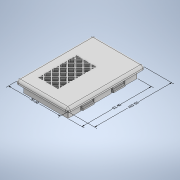
# Autodesk Inventor part: Part_A2
Saved by Autodesk Inventor 2022.6 (Build 266554010, 554A)
## iProperties
Created: 2025-05-14
Part Number: Part_A2
Material: Generic
Document SubType Name: Modeling
Designer: khinm
Density: 1 g/cm^3
Appearance: Default
Author: khinm
Autodesk Inventor part; units mm, degrees
ref_plane "YZ Plane" through (0, 0, 0) normal (1, 0, 0) x (0, 1, 0)
ref_plane "XZ Plane" through (0, 0, 0) normal (0, 1, 0) x (-1, 0, 0)
sketch "Sketch1" plane through (0, 0, 0) normal (0, 1, 0) x (-1, 0, 0)
  line L0 (35, -51.75) -> (-35, -51.75)
  line L1 (-35, -51.75) -> (-35, 51.75)
  line L2 (-35, 51.75) -> (35, 51.75)
  line L3 (35, 51.75) -> (35, -51.75)
  point P0 (0, 0)
  point P1 (35, 0)
  point P2 (0, -51.75)
  dimension "d0" = 70
  dimension "d1" = 103.5
  constraints: 8 end point, 2 midpoint, 2 parallel, 1 horizontal, 1 horizontal alignment, 1 perpendicular, 1 vertical alignment
  measures "d0" distance of L0.start L0.end
  measures "d1" distance of L0.end L1.end
extrude "Extrusion1" add sketch "Sketch1" along normal blind 5
sketch "Sketch2" plane through (0, 0, 0) normal (0, -1, 0) x (1, 0, 0)
  line L0 (-29.95, 46.7) -> (29.95, 46.7)
  line L1 (29.95, 46.7) -> (29.95, -46.7)
  line L2 (29.95, -46.7) -> (-29.95, -46.7)
  line L3 (-29.95, -46.7) -> (-29.95, 46.7)
  line L4 (-35, -51.75) -> (-35, 51.75) projected
  line L5 (-35, 51.75) -> (35, 51.75) projected
  point P0 (0, 0)
  point P1 (-29.95, 0)
  point P2 (-35, 0)
  point P3 (0, 46.7)
  point P4 (0, 51.75)
  dimension "d4" = 59.9
  dimension "d5" = 93.4
  constraints: 8 end point, 4 midpoint, 2 parallel, 1 horizontal, 1 horizontal alignment, 1 perpendicular, 1 vertical alignment
  measures "d4" distance of L0.start L0.end
  measures "d5" distance of L0.end L1.end
extrude "Extrusion2" add sketch "Sketch2" along normal blind 11
sketch "Sketch3" plane through (0, -11, 0) normal (0, -1, 0) x (1, 0, 0)
  line L0 (-28.45, 45.2) -> (28.45, 45.2)
  line L1 (28.45, 45.2) -> (28.45, -45.2)
  line L2 (28.45, -45.2) -> (-28.45, -45.2)
  line L3 (-28.45, -45.2) -> (-28.45, 45.2)
  line L4 (29.95, 46.7) -> (-29.95, 46.7) projected
  line L5 (-29.95, 46.7) -> (-29.95, -46.7) projected
  point P0 (0, 0)
  point P1 (0, 45.2)
  point P2 (0, 46.7)
  point P3 (-28.45, 0)
  dimension "d8" = 1.5
  dimension "d9" = 1.5
  constraints: 8 end point, 3 midpoint, 2 parallel, 2 vertical alignment, 1 horizontal, 1 horizontal alignment, 1 perpendicular
  measures "d8" distance between parallel lines of L4 L0
  measures "d9" distance between parallel lines of L5 L3
extrude "Extrusion3" cut sketch "Sketch3" against normal up to surface (11 mm away)
sketch "Sketch4" plane through (29.95, 0, 46.7) normal (1, 0, 0) x (0, 0, -1)
  line L0 (93.4, -11) -> (0, -11) projected
  line L1 (17.025, -2) -> (18.525, -2)
  line L2 (18.525, -2) -> (18.525, -11)
  line L3 (18.525, -11) -> (17.025, -11)
  line L4 (17.025, -11) -> (17.025, -2)
  line L5 (58.375, -2) -> (59.875, -2)
  line L6 (59.875, -2) -> (59.875, -11)
  line L7 (59.875, -11) -> (58.375, -11)
  line L8 (58.375, -11) -> (58.375, -2)
  line L9 (33.525, -2) -> (35.025, -2)
  line L10 (35.025, -2) -> (35.025, -11)
  line L11 (35.025, -11) -> (33.525, -11)
  line L12 (33.525, -11) -> (33.525, -2)
  line L13 (74.875, -2) -> (76.375, -2)
  line L14 (76.375, -2) -> (76.375, -11)
  line L15 (76.375, -11) -> (74.875, -11)
  line L16 (74.875, -11) -> (74.875, -2)
  line L17 (35.025, -11) -> (58.375, -11)
  line L18 (-5.05, 0) -> (98.45, 0) projected
  point P0 (46.7, 0)
  point P1 (46.7, 0)
  point P2 (46.7, -11)
  point P3 (17.025, -11)
  dimension "d12" = 1.5
  dimension "d13" = 9
  dimension "d14" = 1.5
  dimension "d15" = 9
  dimension "d16" = 9
  dimension "d17" = 1.5
  dimension "d18" = 1.5
  dimension "d19" = 23.35
  dimension "d20" = 15
  dimension "d21" = 15
  constraints: 34 end point, 8 parallel, 5 point on line, 4 horizontal, 4 perpendicular, 2 midpoint, 1 collinear, 1 vertical alignment
  measures "d12" distance of L1.start L1.end
  measures "d13" distance of L1.end L2.end
  measures "d14" distance between parallel lines of L6 L8
  measures "d15" distance of L9.end L10.end
  measures "d16" distance of L13.end L14.end
  measures "d17" distance between parallel lines of L10 L12
  measures "d18" distance between parallel lines of L14 L16
  measures "d19" distance between parallel lines of L8 L10
  measures "d20" distance between parallel lines of L2 L12
  measures "d21" distance between parallel lines of L16 L6
extrude "Extrusion4" cut sketch "Sketch4" against normal up to surface (1.5 mm away)
mirror "Mirror1" about plane through (0, 0, 0) normal (1, 0, 0) of "Extrusion4"
ref_plane "Work Plane1" through (0, 0, 28.175) normal (0, 0, 1) x (1, 0, 0)
sketch "Sketch6" plane through (0, 0, 28.175) normal (0, 0, 1) x (1, 0, 0)
  line L0 (-29.95, -11) -> (29.95, -11) projected
  line L1 (29.95, -11) -> (29.95, -2) projected
  line L2 (-29.95, -2) -> (-29.95, -11) projected
  line L3 (29.95, -11) -> (31.95, -10)
  line L4 (31.95, -10) -> (31.95, -8.1)
  line L5 (31.95, -8.1) -> (29.95, -7.1)
  line L6 (29.95, -11) -> (29.95, -2) projected
  line L7 (29.95, -7.1) -> (29.95, -11)
  point P0 (0, 0)
  point P1 (29.95, -9.05)
  point P2 (31.95, -9.05)
  dimension "d25" = 2
  dimension "d26" = 3.9
  dimension "d27" = 1.9
  constraints: 8 end point, 2 midpoint, 1 equal length, 1 parallel, 1 point on line, 1 vertical
  measures "d25" distance of point (29.95, -9.05) point (31.95, -9.05)
  measures "d26" distance of L0.end L5.end
  measures "d27" distance of L3.end L4.end
extrude "Extrusion5" add sketch "Sketch6" against normal up to surface (15 mm away)
mirror "Mirror2" about plane through (0, 0, 0) normal (1, 0, 0) of "Extrusion5"
mirror "Mirror3" about plane through (0, 0, 0) normal (0, 0, 1) of "Extrusion5", "Mirror2"
fillet "Fillet1" radius 3 8 edges at (35, 5, 0) (0, 5, 51.75) (-35, 5, 0) (0, 5, -51.75) (35, 2.5, -51.75) (35, 2.5, 51.75) (-35, 2.5, 51.75) (-35, 2.5, -51.75)
fillet "Fillet2" radius 0.5 4 edges at (29.95, -5.5, 46.7) (-29.95, -5.5, 46.7) (29.95, -5.5, -46.7) (-29.95, -5.5, -46.7)
sketch "Sketch7" plane through (0, 5, 0) normal (0, 1, 0) x (1, 0, 0)
  line L0 (-21.45, 16.3) -> (4.55, 16.3)
  line L1 (4.55, 16.3) -> (4.55, -34.7)
  line L2 (4.55, -34.7) -> (-21.45, -34.7)
  line L3 (-21.45, -34.7) -> (-21.45, 16.3)
  line L4 (-0.45, -34.7) -> (2.1566, -32.0934)
  line L5 (3.9244, -30.3256) -> (4.55, -29.7)
  line L6 (-3.1467, -33.8612) -> (0.3888, -30.3256)
  line L7 (2.1566, -28.5579) -> (4.55, -26.1645)
  line L8 (4.55, -30.9513) -> (3.9244, -30.3256)
  line L9 (4.55, -34.4868) -> (2.1566, -32.0934)
  line L10 (2.1566, -28.5579) -> (-1.3789, -25.0223)
  line L11 (0.3888, -30.3256) -> (-3.1467, -26.7901)
  line L12 (-3.1467, -33.8612) -> (-6.6822, -30.3256)
  line L13 (-13.7533, -33.8612) -> (-10.2178, -30.3256)
  line L14 (-8.45, -28.5579) -> (-4.9145, -25.0223)
  line L15 (-5.8434, -34.7) -> (-8.45, -32.0934)
  line L16 (-11.0566, -34.7) -> (-8.45, -32.0934)
  line L17 (-6.6822, -30.3256) -> (-3.1467, -26.7901)
  line L18 (-21.45, -34.4868) -> (-19.0566, -32.0934)
  line L19 (-21.45, -30.9513) -> (-20.8244, -30.3256)
  line L20 (-16.45, -34.7) -> (-19.0566, -32.0934)
  line L21 (-20.8244, -30.3256) -> (-21.45, -29.7)
  line L22 (-13.7533, -33.8612) -> (-17.2888, -30.3256)
  line L23 (-19.0566, -28.5579) -> (-21.45, -26.1645)
  line L24 (-19.0566, -28.5579) -> (-15.5211, -25.0223)
  line L25 (-17.2888, -30.3256) -> (-13.7533, -26.7901)
  line L26 (-10.2178, -30.3256) -> (-13.7533, -26.7901)
  line L27 (-8.45, -28.5579) -> (-11.9855, -25.0223)
  line L28 (-21.45, -23.8802) -> (-19.0566, -21.4868)
  line L29 (-21.45, -20.3447) -> (-20.8244, -19.719)
  line L30 (-13.7533, -23.2546) -> (-17.2888, -19.719)
  line L31 (-19.0566, -17.9513) -> (-21.45, -15.5579)
  line L32 (-15.5211, -25.0223) -> (-19.0566, -21.4868)
  line L33 (-20.8244, -19.719) -> (-21.45, -19.0934)
  line L34 (-19.0566, -17.9513) -> (-15.5211, -14.4157)
  line L35 (-17.2888, -19.719) -> (-13.7533, -16.1835)
  line L36 (-13.7533, -23.2546) -> (-10.2178, -19.719)
  line L37 (-11.9855, -25.0223) -> (-8.45, -21.4868)
  line L38 (-3.1467, -23.2546) -> (-6.6822, -19.719)
  line L39 (-8.45, -17.9513) -> (-11.9855, -14.4157)
  line L40 (-4.9145, -25.0223) -> (-8.45, -21.4868)
  line L41 (-10.2178, -19.719) -> (-13.7533, -16.1835)
  line L42 (-6.6822, -19.719) -> (-3.1467, -16.1835)
  line L43 (-8.45, -17.9513) -> (-4.9145, -14.4157)
  line L44 (-3.1467, -23.2546) -> (0.3888, -19.719)
  line L45 (2.1566, -17.9513) -> (4.55, -15.5579)
  line L46 (-1.3789, -25.0223) -> (2.1566, -21.4868)
  line L47 (3.9244, -19.719) -> (4.55, -19.0934)
  line L48 (4.55, -20.3447) -> (3.9244, -19.719)
  line L49 (2.1566, -17.9513) -> (-1.3789, -14.4157)
  line L50 (4.55, -23.8802) -> (2.1566, -21.4868)
  line L51 (0.3888, -19.719) -> (-3.1467, -16.1835)
  line L52 (-21.45, -13.2736) -> (-19.0566, -10.8802)
  line L53 (-21.45, -9.7381) -> (-20.8244, -9.1124)
  line L54 (-13.7533, -12.648) -> (-17.2888, -9.1124)
  line L55 (-19.0566, -7.3447) -> (-21.45, -4.9513)
  line L56 (-15.5211, -14.4157) -> (-19.0566, -10.8802)
  line L57 (-20.8244, -9.1124) -> (-21.45, -8.4868)
  line L58 (-19.0566, -7.3447) -> (-15.5211, -3.8091)
  line L59 (-17.2888, -9.1124) -> (-13.7533, -5.5769)
  line L60 (-13.7533, -12.648) -> (-10.2178, -9.1124)
  line L61 (-11.9855, -14.4157) -> (-8.45, -10.8802)
  line L62 (-3.1467, -12.648) -> (-6.6822, -9.1124)
  line L63 (-8.45, -7.3447) -> (-11.9855, -3.8091)
  line L64 (-4.9145, -14.4157) -> (-8.45, -10.8802)
  line L65 (-10.2178, -9.1124) -> (-13.7533, -5.5769)
  line L66 (4.55, -13.2736) -> (2.1566, -10.8802)
  line L67 (-1.3789, -14.4157) -> (2.1566, -10.8802)
  line L68 (3.9244, -9.1124) -> (4.55, -8.4868)
  line L69 (-3.1467, -12.648) -> (0.3888, -9.1124)
  line L70 (2.1566, -7.3447) -> (4.55, -4.9513)
  line L71 (4.55, -9.7381) -> (3.9244, -9.1124)
  line L72 (-21.45, -2.667) -> (-19.0566, -0.2736)
  line L73 (-15.5211, -3.8091) -> (-19.0566, -0.2736)
  line L74 (-20.8244, 1.4942) -> (-21.45, 2.1198)
  line L75 (-21.45, 0.8685) -> (-20.8244, 1.4942)
  line L76 (-13.7533, -2.0414) -> (-17.2888, 1.4942)
  line L77 (-19.0566, 3.2619) -> (-21.45, 5.6553)
  line L78 (-21.45, 7.9396) -> (-19.0566, 10.333)
  line L79 (-17.2888, 12.1008) -> (-13.7533, 15.6363)
  line L80 (-21.45, 11.4751) -> (-20.8244, 12.1008)
  line L81 (-19.0566, 13.8685) -> (-16.6251, 16.3)
  line L82 (-19.0566, 13.8685) -> (-21.45, 16.2619)
  line L83 (-20.8244, 12.1008) -> (-21.45, 12.7264)
  line L84 (-8.45, 13.8685) -> (-10.8815, 16.3)
  line L85 (-8.45, 13.8685) -> (-6.0185, 16.3)
  line L86 (-6.6822, 12.1008) -> (-3.1467, 15.6363)
  line L87 (-10.2178, 12.1008) -> (-13.7533, 15.6363)
  line L88 (-13.7533, 8.5652) -> (-17.2888, 12.1008)
  line L89 (-19.0566, 3.2619) -> (-15.5211, 6.7975)
  line L90 (-13.7533, 8.5652) -> (-10.2178, 12.1008)
  line L91 (-15.5211, 6.7975) -> (-19.0566, 10.333)
  line L92 (-17.2888, 1.4942) -> (-13.7533, 5.0297)
  line L93 (-11.9855, 6.7975) -> (-8.45, 10.333)
  line L94 (-13.7533, -2.0414) -> (-10.2178, 1.4942)
  line L95 (-8.45, 3.2619) -> (-11.9855, 6.7975)
  line L96 (-11.9855, -3.8091) -> (-8.45, -0.2736)
  line L97 (-10.2178, 1.4942) -> (-13.7533, 5.0297)
  line L98 (-4.9145, 6.7975) -> (-8.45, 10.333)
  line L99 (-8.45, 3.2619) -> (-4.9145, 6.7975)
  line L100 (-6.6822, 1.4942) -> (-3.1467, 5.0297)
  line L101 (-3.1467, 8.5652) -> (-6.6822, 12.1008)
  line L102 (4.55, 7.9396) -> (2.1566, 10.333)
  line L103 (0.3888, 12.1008) -> (-3.1467, 15.6363)
  line L104 (-3.1467, 8.5652) -> (0.3888, 12.1008)
  line L105 (2.1566, 13.8685) -> (4.55, 16.2619)
  line L106 (-1.3789, 6.7975) -> (2.1566, 10.333)
  line L107 (3.9244, 12.1008) -> (4.55, 12.7264)
  line L108 (4.55, 11.4751) -> (3.9244, 12.1008)
  line L109 (2.1566, 13.8685) -> (-0.2749, 16.3)
  line L110 (2.1566, 3.2619) -> (4.55, 5.6553)
  line L111 (4.55, -2.667) -> (2.1566, -0.2736)
  line L112 (0.3888, 1.4942) -> (-3.1467, 5.0297)
  line L113 (4.55, 0.8685) -> (3.9244, 1.4942)
  line L114 (2.1566, 3.2619) -> (-1.3789, 6.7975)
  line L115 (3.9244, 1.4942) -> (4.55, 2.1198)
  line L116 (-6.6822, -9.1124) -> (-3.1467, -5.5769)
  line L117 (-1.3789, -3.8091) -> (2.1566, -0.2736)
  line L118 (-8.45, -7.3447) -> (-4.9145, -3.8091)
  line L119 (-3.1467, -2.0414) -> (0.3888, 1.4942)
  line L120 (0.3888, -9.1124) -> (-3.1467, -5.5769)
  line L121 (-4.9145, -3.8091) -> (-8.45, -0.2736)
  line L122 (2.1566, -7.3447) -> (-1.3789, -3.8091)
  line L123 (-3.1467, -2.0414) -> (-6.6822, 1.4942)
  point P0 (0, 0)
  point P1 (29.45, -46.7)
  point P2 (-29.45, -46.7)
  dimension "d34" = 26
  dimension "d32" = 12
  dimension "d33" = 51
  dimension "d35" = 8
  dimension "d53" = 5
  dimension "d67" = 5
  constraints: 285 parallel, 244 end point, 4 point on line, 2 horizontal, 26 other
  measures "d32" vertical distance of L2.start point (29.45, -46.7)
  measures "d33" distance of L0.end L2.start
  measures "d53" distance of L2.start L5.end
  measures "d67" distance of L4.start L2.start
extrude "Extrusion6" cut sketch "Sketch7" against normal up to surface (5 mm away) contours L0 L81 L82 L3 | L0 L85 L84 | L83 L80 L3 | L0 L1 L105 L109 | L78 L91 L89 L77 L3 | L74 L75 L3 | L1 L108 L107 | L72 L73 L58 L55 L3 | L1 L110 L114 L106 L102 | L57 L53 L3 | L1 L113 L115 | L52 L56 L34 L31 L3 | L1 L70 L122 L117 L111 | L33 L29 L3 | L1 L71 L68 | L28 L32 L24 L23 L3 | L1 L45 L49 L67 L66 | L21 L19 L3 | L1 L48 L47 | L18 L20 L2 L3 | L1 L7 L10 L46 L50 | L1 L8 L5 | L16 L15 L2 | L1 L2 L4 L9 | L12 L17 L11 L6 | L22 L25 L26 L13 | L27 L37 L40 L14 | L30 L35 L41 L36 | L38 L42 L51 L44 | L39 L61 L64 L43 | L54 L59 L65 L60 | L62 L116 L120 L69 | L63 L96 L121 L118 | L76 L92 L97 L94 | L79 L87 L90 L88 | L86 L103 L104 L101 | L93 L98 L99 L95 | L100 L112 L119 L123
chamfer "Chamfer1" distance 0.5 angle 45 120 edges at (0.3888, 5, 12.648) (0.3888, 5, 16.1835) (3.3533, 5, 12.0769) (-1.3789, 5, 7.3447) (-4.9145, 5, 10.8802) (-4.9145, 5, 7.3447) (-1.3789, 5, 10.8802) (-10.2178, 5, 5.5769) (-10.2178, 5, 2.0414) (-6.6822, 5, 2.0414) (-6.6822, 5, 5.5769) (-15.5211, 5, 0.2736) (-15.5211, 5, -3.2619) (-11.9855, 5, -3.2619) (-11.9855, 5, 0.2736) (-6.6822, 5, -5.0297) (-10.2178, 5, -8.5652) (-6.6822, 5, -8.5652) (-10.2178, 5, -5.0297) (-11.9855, 5, -10.333) (-11.9855, 5, -13.8685) (-7.2343, 5, -15.0843) (-9.6657, 5, -15.0843) (-4.9145, 5, -10.333) (-1.3789, 5, -13.8685) (-4.9145, 5, -13.8685) (-1.3789, 5, -10.333) (0.3888, 5, -8.5652) (3.3533, 5, -9.1363) (3.3533, 5, -4.4586) (0.3888, 5, -5.0297) (-1.3789, 5, -3.2619) (-4.9145, 5, -3.2619) (-4.9145, 5, 0.2736) (-1.3789, 5, 0.2736) (0.3888, 5, 2.0414) (0.3888, 5, 5.5769) (3.3533, 5, 1.4703) (3.3533, 5, 6.148) (4.2372, 5, -1.807) (4.2372, 5, -1.1814) (4.2372, 5, -11.788) (4.2372, 5, -12.4136) (3.3533, 5, -15.0652) (0.9409, 5, -15.0843) (-17.8409, 5, -15.0843) (-20.2533, 5, -15.0652) (-21.1372, 5, -11.788) (-21.1372, 5, -12.4136) (-20.2533, 5, -9.1363) (-17.2888, 5, -8.5652) (-15.5211, 5, -10.333) (-15.5211, 5, -13.8685) (-17.2888, 5, -5.0297) (-20.2533, 5, -4.4586) (-21.1372, 5, -1.807) (-21.1372, 5, -1.1814) (-20.2533, 5, 1.4703) (-17.2888, 5, 2.0414) (-15.5211, 5, 7.3447) (-17.2888, 5, 5.5769) (-20.2533, 5, 6.148) (-21.1372, 5, 8.7996) (-21.1372, 5, 9.4252) (-20.2533, 5, 12.0769) (-17.2888, 5, 12.648) (-15.5211, 5, 10.8802) (-11.9855, 5, 10.8802) (-10.2178, 5, 12.648) (-11.9855, 5, 7.3447) (-6.6822, 5, 12.648) (-6.6822, 5, 16.1835) (-10.2178, 5, 16.1835) (-17.2888, 5, 16.1835) (-15.5211, 5, 17.9513) (-11.9855, 5, 21.4868) (-11.9855, 5, 17.9513) (-15.5211, 5, 21.4868) (-20.2533, 5, 16.7546) (-21.1372, 5, 19.4062) (-21.1372, 5, 20.0318) (-4.9145, 5, 21.4868) (-4.9145, 5, 17.9513) (-1.3789, 5, 17.9513) (-1.3789, 5, 21.4868) (3.3533, 5, 16.7546) (4.2372, 5, 9.4252) (4.2372, 5, 8.7996) (-20.2533, 5, 22.6835) (-20.2533, 5, 27.3612) (-17.2888, 5, 23.2546) (-17.2888, 5, 26.7901) (-17.7533, 5, 33.3967) (-20.2533, 5, 33.2901) (-21.1372, 5, 30.0128) (-21.1372, 5, 30.6384) (-15.5211, 5, 32.0934) (-15.5211, 5, 28.5579) (-11.9855, 5, 28.5579) (-11.9855, 5, 32.0934) (-9.7533, 5, 33.3967) (-7.1467, 5, 33.3967) (-4.9145, 5, 28.5579) (-6.6822, 5, 26.7901) (-10.2178, 5, 23.2546) (-10.2178, 5, 26.7901) (-6.6822, 5, 23.2546) (-1.3789, 5, 28.5579) (-1.3789, 5, 32.0934) (-4.9145, 5, 32.0934) (0.8533, 5, 33.3967) (3.3533, 5, 33.2901) (3.3533, 5, 27.3612) (0.3888, 5, 26.7901) (0.3888, 5, 23.2546) (3.3533, 5, 22.6835) (4.2372, 5, 30.0128) (4.2372, 5, 30.6384) (4.2372, 5, 20.0318) (4.2372, 5, 19.4062)
body "Solid1"
